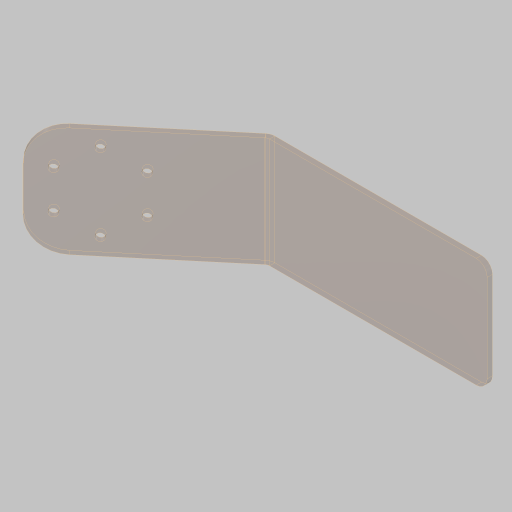
# Autodesk Inventor part: CL7-023
Saved by Autodesk Inventor 2023.5 (Build 275446000, 446)
## iProperties
Created: 2025-04-01
Part Number: CL7-023
Material: Polycarbonate, Smoke
Document SubType Name: Sheet Metal
Designer: slick
Density: 1.2 g/cm^3
Sheet Metal Rule: Default
Appearance: Polycarbonate - Smoked
Author: slick
Autodesk Inventor part; units mm, degrees
ref_plane "YZ Plane" through (0, 0, 0) normal (1, 0, 0) x (0, 1, 0)
ref_plane "XZ Plane" through (0, 0, 0) normal (0, 1, 0) x (-1, 0, 0)
ref_plane "XY Plane" through (0, 0, 0) normal (0, 0, 1) x (1, 0, 0)
sketch "Sketch1" plane through (0, 0, 0) normal (0, 0, 1) x (1, 0, 0)
  line L0 (63.5, -31.75) -> (-63.5, -31.75)
  line L1 (-63.5, -31.75) -> (-63.5, 31.75)
  line L2 (-63.5, 31.75) -> (63.5, 31.75)
  line L3 (63.5, 31.75) -> (63.5, -31.75)
  line L4 (63.5, -31.75) -> (-63.5, 31.75) construction
  line L5 (-63.5, -31.75) -> (63.5, 31.75) construction
  point P0 (0, 0)
  dimension "d0" = 63.5
  dimension "d1" = 127
  measures "d0" distance between parallel lines of L2 L0
  measures "d1" distance of L1.end L2.end
extrude "Plate1" add sketch "Sketch1" along normal blind 3.048
sketch "Sketch2" plane through (-63.5, -31.75, 3.048) normal (-0.6427876, 0, -0.7660444) x (0, -1, 0)
  line L0 (-63.5, 0) -> (0, 0)
  line L1 (0, 0) -> (0, 100.4906)
  line L2 (0, 100.4906) -> (-63.5, 100.4906)
  line L3 (-63.5, 100.4906) -> (-63.5, 0)
  constraints: 6 end point, 1 horizontal, 1 perpendicular, 1 vertical
edge flange "Flange1" height 101.6 angle 40 thickness 3.048 bend radius 3.048 thickness toward (-0.6427876, 0, -0.7660444) relief tear relief width 3.048 relief depth 1.524 edges at (-63.5, 0, 3.048) wall of the first edge with corners at (-63.5, 31.75, 3.048) (-63.5, -31.75, 3.048) (-140.4803, -31.75, 67.6421) (-140.4803, 31.75, 67.6421)
bend "Bend1"
corner "Corner1"
sketch "Sketch3" plane through (-142.4395, -31.75, 65.3072) normal (-0.6427876, 0, -0.7660444) x (-0.7660444, 0, 0.6427876)
  circle A0 centre (-31.75, 31.75) radius 22.225 construction
  line L0 (-99.3812, 63.5) -> (0, 63.5) construction
  line L1 (0, 63.5) -> (0, 0) construction
  point P0 (-151.0937, 31.75)
  point P1 (-49.6906, 63.5)
  point P2 (-31.75, 53.975)
  point P3 (-50.9974, 42.8625)
  point P4 (-50.9974, 20.6375)
  point P5 (-31.75, 9.525)
  point P6 (-12.5026, 20.6375)
  point P7 (-12.5026, 42.8625)
  dimension "d13" = 44.45
  dimension "d16" = 360
  dimension "d25" = 31.75
  constraints: 2 vertical alignment, 1 horizontal alignment, 1 midpoint, 9 other
  measures "d25" distance from line of L1 point (-31.75, 31.75)
hole "Hole1" at (-118.1176, 22.225, 44.8987) at (-103.3732, 11.1125, 32.5267) at (-103.3732, -11.1125, 32.5267) at (-118.1176, -22.225, 44.8987) at (-132.862, -11.1125, 57.2707) at (-132.862, 11.1125, 57.2707) direction (0.6427876, 0, 0.7660444) diameter 4.4958 depth 3.048 tip angle 118 clearance for "Flat Head Machine Screw (82)" size "#8" standard "Ansi Unified Screw Threads"
fillet "Fillet1" radius 19.05 2 edges at (-141.4599, -31.75, 66.4747) (-141.4599, 31.75, 66.4747)
fillet "Fillet2" radius 6.35 2 edges at (63.5, 31.75, 1.524) (63.5, -31.75, 1.524)
equation "\"d23\" = Thickness"
equation "\"d2\" = Thickness"
equation "\"d3\" = BendReliefWidth"
equation "\"d4\" = BendReliefDepth"
equation "\"d5\" = MinimumRemnant"
equation "\"d6\" = TransitionRadius"
equation "\"d9\" = BendRadius"
equation "\"d10\" = CornerReliefSize"
equation "\"d11\" = GapSize"
equation "\"d12\" = JacobiRadiusSize"
equation "\"BendRadius\" = Thickness"
equation "\"BendReliefWidth\" = Thickness"
equation "\"BendReliefDepth\" = 0.5 * Thickness"
equation "\"CornerReliefSize\" = 4 * Thickness"
equation "\"MinimumRemnant\" = 2 * Thickness"
equation "\"TransitionRadius\" = BendRadius"
equation "\"JacobiRadiusSize\" = BendRadius"
equation "\"GapSize\" = Thickness"
equation "\"Thickness\" = 3.048"
body "Solid1"
